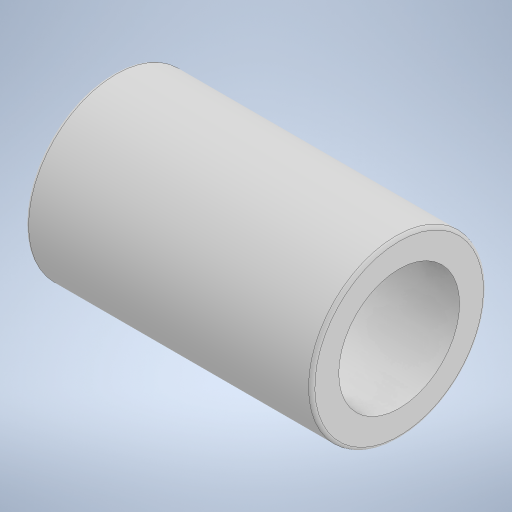
# Autodesk Inventor part: linker
Saved by Autodesk Inventor 2023 (Build 270158000, 158)
## iProperties
Created: 2023-03-19
Part Number: linker
Material: Generic
Document SubType Name: Modeling
Designer: forti
Density: 1 g/cm^3
Appearance: Default
Author: forti
Autodesk Inventor part; units mm, degrees
ref_plane "YZ Plane" through (0, 0, 0) normal (1, 0, 0) x (0, 1, 0)
ref_plane "XZ Plane" through (0, 0, 0) normal (0, 1, 0) x (-1, 0, 0)
ref_plane "XY Plane" through (0, 0, 0) normal (0, 0, 1) x (1, 0, 0)
sketch "Sketch1" plane through (0, 0, 0) normal (0, 1, 0) x (-1, 0, 0)
  point P0 (0, 0)
sketch "Sketch2" plane through (0, 0, 0) normal (0, 1, 0) x (-1, 0, 0)
  line L0 (29.6036, 0) -> (-33.9054, 0)
  circle A0 centre (0, -19) radius 1.5
  point P0 (0, 0)
  dimension "d0" = 19
  dimension "d1" = 3
  constraints: 2 end point, 1 centre point, 1 coincident, 1 horizontal
  measures "d0" distance from line of L0 point (0, -19)
  measures "d1" diameter of A0
revolve "Revolution1" add sketch "Sketch2" angle 360 about axis through (-29.6036, 0, 0) along (1, 0, 0)
sketch "Sketch3" plane through (0, 0, 0) normal (1, 0, 0) x (0, 1, 0)
  circle A0 centre (0, 0) radius 19
  circle A1 centre (0, 0) radius 27.5
  dimension "d3" = 38
  dimension "d4" = 55
  constraints: 2 centre point, 2 coincident
  measures "d3" diameter of A0
  measures "d4" diameter of A1
extrude "Extrusion1" add sketch "Sketch3" along normal mid plane 90
fillet "Fillet1" radius 1 1 edges at (45, -27.5, 0)
fillet "Fillet2" radius 1 1 edges at (-45, -27.5, 0)
body "Solid1"
